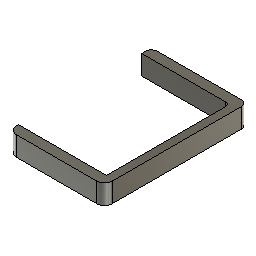
cclump (Autodesk Fusion 360 design; units mm, degrees)
Autodesk Fusion 360 part; units mm, degrees
sketch "Sketch1" plane through (0, 0, 0) normal (0, 0, 1) x (1, 0, 0) in component "Component"
  line L0 (0, 0) -> (45, 0)
  line L1 (45, 0) -> (45, 63)
  line L2 (45, 63) -> (0, 63)
  line L3 (0, 63) -> (0, 0)
  line L4 (0, 63) -> (0, 65)
  line L5 (3, 68) -> (46, 68)
  line L6 (49, 65) -> (49, -1)
  line L7 (45, -5) -> (4, -5)
  line L8 (0, -1) -> (0, 0)
  arc A0 (49, 65) -> (46, 68) centre (46, 65) ccw
  arc A1 (3, 68) -> (0, 65) centre (3, 65) ccw
  arc A2 (45, -5) -> (49, -1) centre (45, -1) ccw
  arc A3 (0, -1) -> (4, -5) centre (4, -1) ccw
  point P0 (0, 68)
  dimension "d1" = 45
  dimension "d2" = 63
  dimension "d3" = 5
  dimension "d4" = 3
  dimension "d5" = 3
  dimension "d6" = 4
  dimension "d7" = 4
  constraint horizontal L0
  constraint vertical L1
  constraint horizontal L2
  constraint vertical L3
  constraint coincident L0.start L3.end
  constraint perpendicular L2 L4
  constraint perpendicular L4 L5
  constraint perpendicular L5 L6
  constraint perpendicular L6 L7
  constraint perpendicular L0 L8
  constraint tangent L5 A0
  constraint tangent L6 A0
  constraint coincident P0 L4
  constraint coincident P0 L5
  constraint tangent L4 A1
  constraint tangent L5 A1
  constraint tangent L6 A2
  constraint tangent L7 A2
  constraint tangent L7 A3
  constraint tangent L8 A3
  measures "d1" distance of L0.start L0.end
  measures "d2" distance of L0.start L2.end
  measures "d3" distance of L2.end P0
  measures "d4" radius of A0
  measures "d5" radius of A1
  measures "d6" radius of A2
  measures "d7" radius of A3
extrude "Extrude1" add sketch "Sketch1" along normal blind 10 contours L0 L1 L2 L4 L5 L6 L7 L8 A0 A1 A2 A3 in component "Component"
fillet "Fillet1" radius 2 1 edges at (45, 63, 5) in component "Component"
component "Component" placed x (1, 0, 0) y (0, 1, 0) z (0, 0, 1) at (0, 0, 0)
